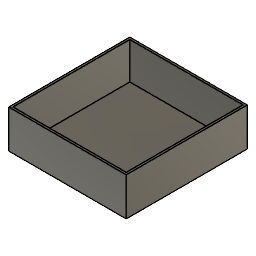
Final Top Bin (Autodesk Fusion 360 design; units mm, degrees)
Autodesk Fusion 360 part; units mm, degrees
note: some values were not read from the file. Set by a fixed rule: which face or edge a step refers to.
sketch "Sketch1" plane through (0, 0, 0) normal (0, 0, 1) x (1, 0, 0)
  line L0 (81.5, 84) -> (-81.5, 84)
  line L1 (-81.5, 84) -> (-81.5, -84)
  line L2 (-81.5, -84) -> (81.5, -84)
  line L3 (81.5, -84) -> (81.5, 84)
  line L4 (81.5, 84) -> (-81.5, -84) construction
  line L5 (-81.5, 84) -> (81.5, -84) construction
  dimension "d3" = 163
  dimension "d4" = 168
  constraint horizontal L0
  constraint perpendicular L0 L1
  constraint parallel L0 L2
  constraint parallel L1 L3
  constraint coincident L4 origin
  constraint coincident L5 origin
  measures "d3" distance of L1.end L2.end
  measures "d4" distance of L0.end L1.end
extrude "Extrude1" add sketch "Sketch1" along normal blind 53
shell "Shell1" thickness 3 removed faces 1 at (27.1667, -28, 53)
move_face "OffsetFaces1" offset 2 1 faces at (26.1667, -27, 3)
extrude "Extrude2" cut 1 faces at (26.1667, -27, 5) along direction (0, 0, -1) blind 3
